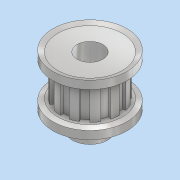
# Autodesk Inventor part: Koło zębate 21 T5 12 2F
Saved by Autodesk Inventor 2018 (Build 220112000, 112)
## iProperties
Created: 2019-01-23
Part Number: Koło zębate 21 T5 12 2F
Material: Ogólny
Document SubType Name: Modeling
Designer: Dawid
Density: 1 g/cm^3
Appearance: Aluminium — ciemne
Author: Dawid
Autodesk Inventor part; units mm, degrees
ref_plane "YZ Plane" through (0, 0, 0) normal (1, 0, 0) x (0, 1, 0)
ref_plane "XZ Plane" through (0, 0, 0) normal (0, 1, 0) x (-1, 0, 0)
ref_plane "XY Plane" through (0, 0, 0) normal (0, 0, 1) x (1, 0, 0)
sketch "Szkic1" plane through (0, 0, 0) normal (0, 0, 1) x (1, 0, 0)
  arc A0 (2.3617, 8.8141) -> (0, 9.125) centre (0, 0) ccw
  arc A1 (0, 8.125) -> (2.1029, 7.8481) centre (0, 0) ccw
  line L0 (0, 0) -> (0, 9.125)
  line L1 (2.1029, 7.8481) -> (2.3617, 8.8141)
  line L2 (0, 0) -> (9.125, 0) construction
  dimension "d0" = 18.25
  dimension "d1" = 16.25
  dimension "d3" = 75
  constraints: 6 end point, 4 point on circle, 2 centre point, 2 coincident, 1 horizontal, 1 point on line, 1 vertical
  measures "d0" diameter of A0
  measures "d1" diameter of A1
  measures "d3" angle of L2 L1
extrude "Wyciągnięcie proste1" add sketch "Szkic1" along normal blind 21
pattern_circular "Szyk kołowy1" count 12 over 360 about axis through (0, 0, 0) along (0, 0, 1) of "Wyciągnięcie proste1"
sketch "Szkic2" plane through (0, 0, 0) normal (0, 0, -1) x (-1, 0, 0)
  line L0 (0, 9.125) -> (0, 8.125) projected
  arc A0 (0, 9.125) -> (-2.3617, 8.8141) centre (0, 0) ccw projected
  line L1 (-2.1029, 7.8481) -> (-2.3617, 8.8141) projected
  arc A1 (-2.1029, 7.8481) -> (-4.0625, 7.0365) centre (0, 0) ccw projected
  line L2 (-4.5625, 7.9025) -> (-4.0625, 7.0365) projected
  arc A2 (-4.5625, 7.9025) -> (-6.4523, 6.4523) centre (0, 0) ccw projected
  line L3 (-5.7452, 5.7452) -> (-6.4523, 6.4523) projected
  arc A3 (-5.7452, 5.7452) -> (-7.0365, 4.0625) centre (0, 0) ccw projected
  line L4 (-7.9025, 4.5625) -> (-7.0365, 4.0625) projected
  arc A4 (-7.9025, 4.5625) -> (-8.8141, 2.3617) centre (0, 0) ccw projected
  line L5 (-7.8481, 2.1029) -> (-8.8141, 2.3617) projected
  arc A5 (-7.8481, 2.1029) -> (-8.125, 0) centre (0, 0) ccw projected
  line L6 (-9.125, 0) -> (-8.125, 0) projected
  arc A6 (-9.125, 0) -> (-8.8141, -2.3617) centre (0, 0) ccw projected
  line L7 (-7.8481, -2.1029) -> (-8.8141, -2.3617) projected
  arc A7 (-7.8481, -2.1029) -> (-7.0365, -4.0625) centre (0, 0) ccw projected
  line L8 (-7.9025, -4.5625) -> (-7.0365, -4.0625) projected
  arc A8 (-7.9025, -4.5625) -> (-6.4523, -6.4523) centre (0, 0) ccw projected
  line L9 (-5.7452, -5.7452) -> (-6.4523, -6.4523) projected
  arc A9 (-5.7452, -5.7452) -> (-4.0625, -7.0365) centre (0, 0) ccw projected
  line L10 (-4.5625, -7.9025) -> (-4.0625, -7.0365) projected
  arc A10 (-4.5625, -7.9025) -> (-2.3617, -8.8141) centre (0, 0) ccw projected
  line L11 (-2.1029, -7.8481) -> (-2.3617, -8.8141) projected
  arc A11 (-2.1029, -7.8481) -> (0, -8.125) centre (0, 0) ccw projected
  line L12 (0, -9.125) -> (0, -8.125) projected
  arc A12 (0, -9.125) -> (2.3617, -8.8141) centre (0, 0) ccw projected
  line L13 (2.1029, -7.8481) -> (2.3617, -8.8141) projected
  arc A13 (2.1029, -7.8481) -> (4.0625, -7.0365) centre (0, 0) ccw projected
  line L14 (4.5625, -7.9025) -> (4.0625, -7.0365) projected
  arc A14 (4.5625, -7.9025) -> (6.4523, -6.4523) centre (0, 0) ccw projected
  line L15 (5.7452, -5.7452) -> (6.4523, -6.4523) projected
  arc A15 (5.7452, -5.7452) -> (7.0365, -4.0625) centre (0, 0) ccw projected
  line L16 (7.9025, -4.5625) -> (7.0365, -4.0625) projected
  arc A16 (7.9025, -4.5625) -> (8.8141, -2.3617) centre (0, 0) ccw projected
  line L17 (7.8481, -2.1029) -> (8.8141, -2.3617) projected
  arc A17 (7.8481, -2.1029) -> (8.125, 0) centre (0, 0) ccw projected
  line L18 (9.125, 0) -> (8.125, 0) projected
  arc A18 (9.125, 0) -> (8.8141, 2.3617) centre (0, 0) ccw projected
  line L19 (7.8481, 2.1029) -> (8.8141, 2.3617) projected
  arc A19 (7.8481, 2.1029) -> (7.0365, 4.0625) centre (0, 0) ccw projected
  line L20 (7.9025, 4.5625) -> (7.0365, 4.0625) projected
  arc A20 (7.9025, 4.5625) -> (6.4523, 6.4523) centre (0, 0) ccw projected
  line L21 (5.7452, 5.7452) -> (6.4523, 6.4523) projected
  arc A21 (5.7452, 5.7452) -> (4.0625, 7.0365) centre (0, 0) ccw projected
  line L22 (4.5625, 7.9025) -> (4.0625, 7.0365) projected
  arc A22 (4.5625, 7.9025) -> (2.3617, 8.8141) centre (0, 0) ccw projected
  line L23 (2.1029, 7.8481) -> (2.3617, 8.8141) projected
  arc A23 (2.1029, 7.8481) -> (0, 8.125) centre (0, 0) ccw projected
  circle A24 centre (0, 0) radius 5.5
  dimension "d9" = 11
  constraints: 1 centre point, 1 coincident
  measures "d9" diameter of A24
extrude "Wyciągnięcie proste2" cut sketch "Szkic2" against normal blind 6
sketch "Szkic3" plane through (0, 0, 0) normal (1, 0, 0) x (0, 1, 0)
  line L0 (0, 18.5) -> (0, 21)
  line L1 (0, 21) -> (0, 18.5)
  line L2 (0, 8.5) -> (0, 6)
  line L3 (0, 6) -> (10, 6)
  line L4 (11.5, 6) -> (11.5, 8)
  line L5 (10, 8.5) -> (0, 8.5)
  line L6 (0, 18.5) -> (10, 18.5)
  line L7 (11.5, 19) -> (11.5, 21)
  line L8 (10, 21) -> (0, 21)
  line L9 (11.5, 6) -> (11.5, 5.5)
  line L10 (10, 6) -> (11.5, 5.5)
  line L11 (11.5, 8) -> (10, 8.5)
  line L12 (11.5, 21) -> (11.5, 21.5)
  line L13 (10, 21) -> (11.5, 21.5)
  line L14 (10, 18.5) -> (11.5, 19)
  point P0 (0, 0)
  dimension "d19" = 11.5
  constraints: 30 end point, 4 perpendicular, 2 horizontal, 2 vertical
  measures "d19" distance of L2.end L4.start
revolve "Obrót1" add sketch "Szkic3" angle 360 about axis through (0, 0, 8.5) along (0, 0, -1)
sketch "Szkic4" plane through (0, 0, 0) normal (0, 0, -1) x (-1, 0, 0)
  circle A0 centre (0, 0) radius 4
  dimension "d31" = 8
  constraints: 1 centre point, 1 coincident
  measures "d31" diameter of A0
extrude "Wyciągnięcie proste3" cut sketch "Szkic4" against normal up to next
